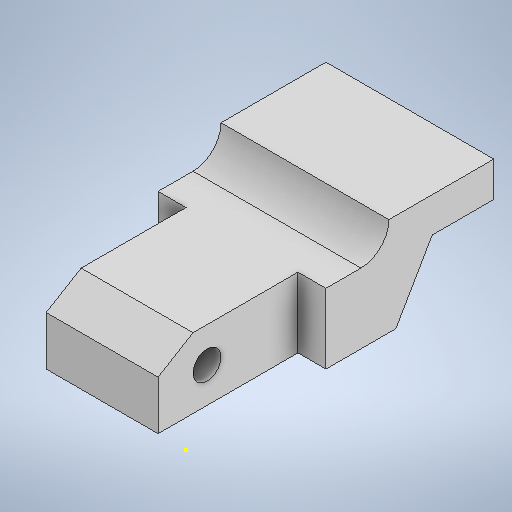
# Autodesk Inventor part: thi1
Saved by Autodesk Inventor 2025.2 (Build 292293000, 293)
## iProperties
Created: 2024-12-05
Part Number: thi1
Material: Generic
Document SubType Name: Modeling
Designer: hongquan
Density: 1 g/cm^3
Appearance: Default
Author: hongquan
Autodesk Inventor part; units mm, degrees
ref_plane "YZ Plane" through (0, 0, 0) normal (1, 0, 0) x (0, 1, 0)
ref_plane "XZ Plane" through (0, 0, 0) normal (0, 1, 0) x (-1, 0, 0)
ref_plane "XY Plane" through (0, 0, 0) normal (0, 0, 1) x (1, 0, 0)
sketch "Sketch1" plane through (0, 0, 0) normal (1, 0, 0) x (0, 1, 0)
  point P0 (0, 0)
sketch "Sketch2" plane through (0, 0, 0) normal (1, 0, 0) x (0, 1, 0)
  line L0 (70, -220) -> (0, -220) construction
  line L1 (0, -220) -> (0, 0) construction
  circle A0 centre (25, -35) radius 10
  line L2 (0, 0) -> (0, -150)
  line L3 (0, -150) -> (161.1976, -150) construction
  line L4 (70, -220) -> (45, -220)
  line L5 (70, -220) -> (70, -145)
  line L6 (70, -145) -> (70, -145)
  line L7 (50, -125) -> (50, 0) construction
  line L8 (50, 0) -> (0, 0) construction
  arc A1 (50, -125) -> (70, -145) centre (70, -125) ccw
  line L9 (50, -25) -> (35, 0)
  line L10 (0, -150) -> (116.4137, -150) construction
  line L11 (45, -220) -> (45, -175.9808)
  line L12 (50, -25) -> (50, -125)
  line L13 (35, 0) -> (0, 0)
  line L14 (0, -150) -> (45, -175.9808)
  point P0 (35, 0)
  point P1 (50, -145)
  point P2 (17.5, 0)
  dimension "d0" = 220
  dimension "d1" = 70
  dimension "d2" = 20
  dimension "d5" = 25
  dimension "d7" = 150
  dimension "d9" = 25
  dimension "d10" = 75
  dimension "d12" = 20
  dimension "d13" = 20
  dimension "d14" = 25
  dimension "d15" = 15
  dimension "d17" = 35
  constraints: 30 end point, 6 point on line, 5 horizontal, 3 tangent, 3 vertical, 2 centre point, 2 point on circle, 1 midpoint, 1 other
  measures "d0" distance of L0.end L1.end
  measures "d1" distance of L0.start L0.end
  measures "d2" diameter of A0
  measures "d5" distance from line of L1 A0.centre
  measures "d7" distance of L1.end L2.end
  measures "d9" distance of L0.start L4.end
  measures "d10" distance of L0.start L5.end
  measures "d12" distance of L5.end point (50, -145)
  measures "d13" radius of A1
  measures "d14" distance from line of L8 L9.start
  measures "d15" distance of L7.end L9.end
  measures "d17" vertical distance of point (17.5, 0) A0.centre
extrude "Extrusion1" add sketch "Sketch2" against normal blind 120
sketch "Sketch3" plane through (0, 70, -145) normal (0, 1, 0) x (1, 0, 0)
  line L0 (0, -145) -> (-120, -145) projected
  line L1 (-60, -145) -> (-60, 75)
  line L2 (0, 75) -> (-120, 75) projected
  line L3 (-120, -145) -> (-120, 75)
  line L4 (-120, 75) -> (0, 75)
  line L5 (0, -145) -> (-120, -145)
  line L6 (0, -145) -> (0, 75)
  line L7 (-100, -145) -> (-20, -145)
  line L8 (-20, -145) -> (-20, -45)
  line L9 (0, 30.9808) -> (-120, 30.9808) projected
  line L10 (-100, -145) -> (-100, -45)
  line L11 (-100, -45) -> (-120, -45)
  line L12 (-20, -45) -> (0, -45)
  dimension "d21" = 80
  dimension "d22" = 100
  constraints: 20 end point, 4 point on line, 3 midpoint, 3 perpendicular, 2 equal length, 1 collinear, 1 horizontal, 1 symmetric about line, 1 vertical
  measures "d21" distance of L7.start L7.end
  measures "d22" distance of L7.end L8.end
extrude "Extrusion2" cut sketch "Sketch3" against normal blind 120 contours L0 L8 L12 L6 | L0 L3 L11 L10
body "Solid1"
